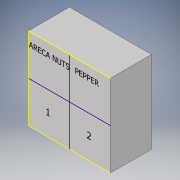
# Autodesk Inventor part: Button
Saved by Autodesk Inventor 2019 (Build 230136000, 136)
## iProperties
Created: 2019-10-19
Part Number: Button
Material: Generic
Document SubType Name: Modeling
Designer: sudhanva
Density: 1 g/cm^3
Appearance: Default
Author: sudhanva
Autodesk Inventor part; units mm, degrees
ref_plane "YZ Plane" through (0, 0, 0) normal (1, 0, 0) x (0, 1, 0)
ref_plane "XZ Plane" through (0, 0, 0) normal (0, 1, 0) x (-1, 0, 0)
ref_plane "XY Plane" through (0, 0, 0) normal (0, 0, 1) x (1, 0, 0)
sketch "Sketch1" plane through (0, 0, 0) normal (0, 0, 1) x (1, 0, 0)
  line L0 (-20, 20) -> (20, 20)
  line L1 (20, 20) -> (20, -20)
  line L2 (20, -20) -> (-20, -20)
  line L3 (-20, -20) -> (-20, 20)
  point P0 (0, 0)
  dimension "d0" = 40
  dimension "d1" = 40
  dimension "d2" = 20
  dimension "d3" = 20
  constraints: 8 end point, 2 parallel, 1 horizontal, 1 perpendicular
  measures "d0" distance of L1.end L2.end
  measures "d1" distance between parallel lines of L2 L0
  measures "d2" distance from line of point (0, 0) L0
  measures "d3" distance from line of point (0, 0) L3
extrude "Extrusion1" add sketch "Sketch1" along normal mid plane 20
sketch "Sketch2" plane through (0, 0, 10) normal (0, 0, 1) x (1, 0, 0)
  line L0 (20, 20) -> (-20, 20) projected
  line L1 (0, 20) -> (0, 0)
  line L2 (0, 0) -> (20, 0)
  line L3 (20, 0) -> (-20, 0)
  line L4 (-20, 20) -> (-20, -20) projected
  line L5 (-19.7277, 15.8039) -> (0.0697, 15.8039) construction
  line L6 (0.0697, 15.8039) -> (0.0697, 13.2067) construction
  line L7 (0.0697, 13.2067) -> (-19.7277, 13.2067) construction
  line L8 (-19.7277, 13.2067) -> (-19.7277, 15.8039) construction
  line L9 (-11.6622, -8.0655) -> (-9.375, -8.0655) construction
  line L10 (-9.375, -8.0655) -> (-9.375, -11.1233) construction
  line L11 (-9.375, -11.1233) -> (-11.6622, -11.1233) construction
  line L12 (-11.6622, -11.1233) -> (-11.6622, -8.0655) construction
  line L13 (2.6158, 15.9129) -> (14.2953, 15.9129) construction
  line L14 (14.2953, 15.9129) -> (14.2953, 13.4129) construction
  line L15 (14.2953, 13.4129) -> (2.6158, 13.4129) construction
  line L16 (2.6158, 13.4129) -> (2.6158, 15.9129) construction
  line L17 (8.3924, -7.9565) -> (10.6797, -7.9565) construction
  line L18 (10.6797, -7.9565) -> (10.6797, -11.0687) construction
  line L19 (10.6797, -11.0687) -> (8.3924, -11.0687) construction
  line L20 (8.3924, -11.0687) -> (8.3924, -7.9565) construction
  constraints: 6 end point, 2 midpoint, 1 horizontal, 1 vertical, 8 other
sketch "Sketch3" plane through (0, 0, 10) normal (0, 0, 1) x (1, 0, 0)
  line L0 (0, 0) -> (0, -20)
  line L1 (-20, -20) -> (20, -20) projected
  constraints: 2 end point, 1 midpoint
body "Solid1"
